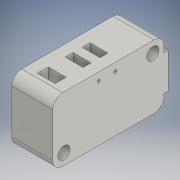
# Autodesk Inventor part: Housing
Saved by Autodesk Inventor 2016 (Build 200138000, 138)
## iProperties
Created: 2016-05-07
Part Number: Housing
Material: ABS Plastic
Document SubType Name: Modeling
Designer: agmle
Density: 1.06 g/cm^3
Appearance: Smooth - White
Author: agmle
Autodesk Inventor part; units mm, degrees
ref_plane "YZ Plane" through (0, 0, 0) normal (1, 0, 0) x (0, 1, 0)
ref_plane "XZ Plane" through (0, 0, 0) normal (0, 1, 0) x (-1, 0, 0)
ref_plane "XY Plane" through (0, 0, 0) normal (0, 0, 1) x (1, 0, 0)
sketch "Sketch1" plane through (0, 0, 0) normal (0, 1, 0) x (-1, 0, 0)
  line L0 (13.5, 13.95) -> (2.5, 13.95)
  line L1 (0, 11.45) -> (0, -11.45)
  line L2 (16, -11.45) -> (16, 11.45)
  line L3 (3.15, -13.95) -> (3.15, -15.03)
  line L4 (3.15, -15.03) -> (12, -15.03)
  line L5 (12, -15.03) -> (12, -13.95)
  line L6 (2.5, -13.95) -> (3.15, -13.95)
  line L7 (12, -13.95) -> (13.5, -13.95)
  arc A0 (16, 11.45) -> (13.5, 13.95) centre (13.5, 11.45) ccw
  arc A1 (2.5, 13.95) -> (0, 11.45) centre (2.5, 11.45) ccw
  arc A2 (0, -11.45) -> (2.5, -13.95) centre (2.5, -11.45) ccw
  arc A3 (13.5, -13.95) -> (16, -11.45) centre (13.5, -11.45) ccw
  point P0 (0, 0)
  point P1 (0, 0)
  dimension "d1" = 16
  dimension "d3" = 8.85
  dimension "d4" = 4
  dimension "d5" = 27.9
  dimension "d6" = 2.5
  dimension "d7" = 1.08
  constraints: 16 end point, 8 point on circle, 8 tangent, 4 centre point, 4 parallel, 3 equal radius, 1 coincident, 1 collinear, 1 horizontal, 1 midpoint, 1 perpendicular
  measures "d1" distance between parallel lines of L1 L2
  measures "d3" distance between parallel lines of L3 L5
  measures "d4" distance between parallel lines of L2 L5
  measures "d5" distance between parallel lines of L0 L7
  measures "d6" radius of A0
  measures "d7" distance between parallel lines of L7 L4
extrude "Extrusion1" add sketch "Sketch1" along normal blind 10.3
sketch "Sketch2" plane through (0, 10.3, 0) normal (0, 1, 0) x (1, 0, 0)
  line L0 (-16, 11.45) -> (-16, -11.45) projected
  line L1 (-12, 13.95) -> (-13.5, 13.95) projected
  line L2 (0, -11.45) -> (0, 11.45) projected
  line L3 (-13.5, -13.95) -> (-2.5, -13.95) projected
  point P0 (0, 0)
  point P1 (-13.2, 11.15)
  point P2 (-2.8, -11.15)
  dimension "d10" = 2.8
  dimension "d11" = 2.8
  dimension "d12" = 2.8
  dimension "d13" = 2.8
  measures "d10" distance from line of L0 point (-13.2, 11.15)
  measures "d11" distance from line of L1 point (-13.2, 11.15)
  measures "d12" distance from line of L2 point (-2.8, -11.15)
  measures "d13" distance from line of L3 point (-2.8, -11.15)
hole "Hole1" at (-13.2, 10.3, -11.15) at (-2.8, 10.3, 11.15) direction (0, -1, 0) diameter 3.1 end through all
sketch "Sketch3" plane through (-16, 0, -11.45) normal (-1, 0, 0) x (0, 0, 1)
  line L0 (10.65, 2.9) -> (8.65, 2.9)
  line L1 (8.65, 2.9) -> (8.65, 7.4)
  line L2 (8.65, 7.4) -> (10.65, 7.4)
  line L3 (10.65, 7.4) -> (10.65, 2.9)
  line L4 (14.9, 2.9) -> (12.9, 2.9)
  line L5 (12.9, 2.9) -> (12.9, 7.4)
  line L6 (12.9, 7.4) -> (14.9, 7.4)
  line L7 (14.9, 7.4) -> (14.9, 2.9)
  line L8 (21.9, 2.9) -> (19.15, 2.9)
  line L9 (19.15, 2.9) -> (19.15, 7.4)
  line L10 (19.15, 7.4) -> (21.9, 7.4)
  line L11 (21.9, 7.4) -> (21.9, 2.9)
  line L12 (25.4, 0) -> (25.4, 10.3) construction
  line L13 (25.4, 5.15) -> (-3.58, 5.15) construction
  line L14 (-3.58, 0) -> (-3.58, 10.3) construction
  point P0 (11.45, 0)
  point P1 (21.9, 5.15)
  point P2 (10.91, 5.15)
  dimension "d21" = 3.5
  dimension "d22" = 2.75
  dimension "d23" = 4.25
  dimension "d24" = 2
  dimension "d25" = 2
  dimension "d26" = 2.25
  dimension "d27" = 4.5
  constraints: 26 end point, 5 parallel, 5 point on line, 4 midpoint, 3 horizontal, 3 perpendicular
  measures "d21" distance between parallel lines of L12 L11
  measures "d22" distance of L8.start L8.end
  measures "d23" distance between parallel lines of L7 L9
  measures "d24" distance of L4.start L4.end
  measures "d25" distance of L0.start L0.end
  measures "d26" distance between parallel lines of L5 L3
  measures "d27" distance of L0.end L1.end
extrude "Extrusion2" cut sketch "Sketch3" against normal blind 3.75
sketch "Sketch4" plane through (0, 10.3, 0) normal (0, 1, 0) x (1, 0, 0)
  line L0 (-16, -3.45) -> (-16, -1.45) construction
  line L1 (-16, -3.45) -> (-12.25, -3.45) construction
  line L2 (-12.25, -3.45) -> (-12.25, -1.45) construction
  line L3 (-16, -1.45) -> (-12.25, -1.45) construction
  line L4 (-16, 0.8) -> (-16, 2.8) construction
  line L5 (-16, 0.8) -> (-12.25, 0.8) construction
  line L6 (-12.25, 0.8) -> (-12.25, 2.8) construction
  line L7 (-16, 2.8) -> (-12.25, 2.8) construction
  line L8 (-14, -2.45) -> (-14, 1.7199) construction
  line L9 (-14, -2.45) -> (-12.25, -2.45) construction
  line L10 (-12.25, -3.45) -> (-12.25, -1.45) construction
  line L11 (-14, 1.7199) -> (-12.25, 1.7199) construction
  line L12 (-12.25, 0.8) -> (-12.25, 2.8) construction
  point P0 (0, 0)
  dimension "d30" = 2
  constraints: 6 end point, 3 perpendicular, 1 midpoint, 1 point on line
  measures "d30" distance between parallel lines of L0 L8
hole "Hole2" at (-14, 10.3, 2.45) at (-14, 10.3, -1.7199) direction (0, -1, 0) diameter 0.75 end through all
equation "\"d11\" = d10"
equation "\"d12\" = d10"
equation "\"d13\" = d10"
body "Solid1"
